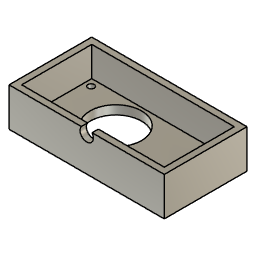
Soporte cámara individual (Parte delantera) (Autodesk Fusion 360 design; units mm, degrees)
Autodesk Fusion 360 part; units mm, degrees
sketch "Boceto1" plane through (0, 0, 0) normal (0, 0, 1) x (1, 0, 0)
  line L0 (-22.6, -11.1) -> (22.6, -11.1)
  line L1 (22.6, -11.1) -> (22.6, 11.1)
  line L2 (22.6, 11.1) -> (-22.6, 11.1)
  line L3 (-22.6, 11.1) -> (-22.6, -11.1)
  line L4 (-22.6, -11.1) -> (22.6, 11.1) construction
  line L5 (22.6, -11.1) -> (-22.6, 11.1) construction
  circle A0 centre (-5.85, 2) radius 8.15
  circle A1 centre (-20.59, 8.89) radius 1
  line L6 (0, 11.1) -> (0, -11.1) construction
  line L7 (22.6, 13.1) -> (-22.6, 13.1)
  line L8 (-22.6, 13.1) -> (-22.6, 11.1)
  line L9 (-22.6, 11.1) -> (22.6, 11.1)
  line L10 (22.6, 11.1) -> (22.6, 13.1)
  line L11 (22.6, 13.1) -> (-22.6, 11.1) construction
  line L12 (-22.6, 13.1) -> (22.6, 11.1) construction
  line L13 (22.6, -13.1) -> (-22.6, -13.1)
  line L14 (-22.6, -13.1) -> (-22.6, -11.1)
  line L15 (-22.6, -11.1) -> (22.6, -11.1)
  line L16 (22.6, -11.1) -> (22.6, -13.1)
  line L17 (22.6, -13.1) -> (-22.6, -11.1) construction
  line L18 (-22.6, -13.1) -> (22.6, -11.1) construction
  line L19 (24.6, -13.1) -> (22.6, -13.1)
  line L20 (22.6, -13.1) -> (22.6, 13.1)
  line L21 (22.6, 13.1) -> (24.6, 13.1)
  line L22 (24.6, 13.1) -> (24.6, -13.1)
  line L23 (24.6, -13.1) -> (22.6, 13.1) construction
  line L24 (22.6, -13.1) -> (24.6, 13.1) construction
  line L25 (-22.6, -13.1) -> (-24.6, -13.1)
  line L26 (-24.6, -13.1) -> (-24.6, 13.1)
  line L27 (-24.6, 13.1) -> (-22.6, 13.1)
  line L28 (-22.6, 13.1) -> (-22.6, -13.1)
  line L29 (-22.6, -13.1) -> (-24.6, 13.1) construction
  line L30 (-24.6, -13.1) -> (-22.6, 13.1) construction
  circle A2 centre (-20.59, -4.89) radius 1
  circle A3 centre (20.59, 8.89) radius 1
  circle A4 centre (20.59, -4.89) radius 1
  point P0 (0, 12.1)
  point P1 (0, -12.1)
  point P2 (23.6, 0)
  point P3 (-23.6, 0)
  dimension "d5" = 22.2
  dimension "d6" = 45.2
  dimension "d7" = 16.3
  dimension "d10" = 2
  dimension "d11" = 2.01
  dimension "d12" = 2.21
  dimension "d13" = 45.2
  dimension "d14" = 2
  dimension "d15" = 45.2
  dimension "d16" = 2
  dimension "d17" = 2
  dimension "d18" = 26.2
  dimension "d19" = 2
  dimension "d20" = 26.2
  dimension "d26" = 16.75
  dimension "d27" = 9.1
  dimension "d28" = 2
  dimension "d29" = 2.01
  dimension "d30" = 6.21
  constraint horizontal L0
  constraint perpendicular L0 L1
  constraint parallel L0 L2
  constraint parallel L1 L3
  constraint coincident L4 origin
  constraint coincident L5 origin
  constraint midpoint L2 L6.start
  constraint midpoint L0 L6.end
  constraint horizontal L7
  constraint perpendicular L7 L8
  constraint parallel L7 L9
  constraint parallel L8 L10
  constraint coincident L11 P0
  constraint coincident L12 P0
  constraint collinear L2 L9
  constraint collinear L3 L8
  constraint horizontal L13
  constraint perpendicular L13 L14
  constraint parallel L13 L15
  constraint parallel L14 L16
  constraint coincident L17 P1
  constraint coincident L18 P1
  constraint collinear L0 L15
  constraint collinear L3 L14
  constraint horizontal L19
  constraint perpendicular L19 L20
  constraint parallel L19 L21
  constraint parallel L20 L22
  constraint coincident L23 P2
  constraint coincident L24 P2
  constraint collinear L1 L20
  constraint collinear L7 L21
  constraint horizontal L25
  constraint perpendicular L25 L26
  constraint parallel L25 L27
  constraint parallel L26 L28
  constraint coincident L29 P3
  constraint coincident L30 P3
  constraint collinear L3 L28
  constraint collinear L7 L27
  constraint symmetric A1 L6 A3
  constraint symmetric L6 A2 A4
  measures "d5" distance of L0.end L1.end
  measures "d6" distance of L1.end L2.end
  measures "d7" diameter of A0
  measures "d10" diameter of A1
  measures "d11" distance of L3 A1.centre
  measures "d12" distance of L2 A1.centre
  measures "d13" distance of L2.end L1.end
  measures "d14" distance of L7.end L2.end
  measures "d15" distance of L0.start L0.end
  measures "d16" distance of L13.end L0.start
  measures "d17" distance of L7.start L21.end
  measures "d18" distance of L13.start L7.start
  measures "d19" distance of L26.end L7.end
  measures "d20" distance of L25.end L26.end
  measures "d26" distance of A0.centre L28
  measures "d27" distance of A0.centre L9
  measures "d28" diameter of A2
  measures "d29" distance of L3 A2.centre
  measures "d30" distance of L0 A2.centre
extrude "Extruir1" add sketch "Boceto1" along normal blind 2.8 contours L0 L1 L2 L3 L9 L15 L20 L28
extrude "Extruir2" add sketch "Boceto1" along normal blind 12.2 contours L3 L8 L14 L25 L26 L27 L28 | L0 L13 L14 L15 L16 L20 L28 | L1 L10 L16 L19 L20 L21 L22 | L2 L7 L8 L9 L10 L20 L28
sketch "Boceto2" plane through (0, -13.1, 0) normal (0, -1, 0) x (1, 0, 0)
  line L0 (-24.6, 0) -> (24.6, 0)
  line L1 (24.6, 0) -> (24.6, 12.2)
  line L2 (24.6, 12.2) -> (-24.6, 12.2)
  line L3 (-24.6, 12.2) -> (-24.6, 0)
  arc A0 (-1.7, 12.2) -> (1.7, 12.2) centre (0, 10.925) ccw
  line L4 (-1.7, 12.2) -> (1.7, 12.2) construction
  line L5 (0, 12.2) -> (0, 8.8) construction
  dimension "d31" = 3.4
  dimension "d32" = 3.4
  constraint coincident L2 A0.end
  constraint coincident L2 A0.start
  constraint midpoint L2 L4
  constraint midpoint L4 L5.start
  constraint midpoint A0 L5.end
  measures "d31" distance of A0.start A0.end
  measures "d32" distance of L5.start L5.end
extrude "Extruir3" cut sketch "Boceto2" against normal blind 2 contours L2 A0
equation "grosor1 = 2.8 mm"
equation "grosor2 = 2 mm"
equation "grosor3 = 7.5 mm"
equation "tolerancia = 0.1 mm"
equation "d5 = 18 mm + tolerancia * 2 + margen_cable"
equation "d6 = 45 mm + tolerancia * 2"
equation "d7 = 16.2 mm + tolerancia"
equation "d10 = 1.9 mm + tolerancia"
equation "d11 = 1.91 mm + tolerancia"
equation "d12 = 2.11 mm + tolerancia"
equation "d13 = d6"
equation "d14 = grosor2"
equation "d15 = d6"
equation "d16 = grosor2"
equation "d17 = grosor2"
equation "d18 = d5 + grosor2 * 2"
equation "d19 = grosor2"
equation "d20 = d5 + grosor2 * 2"
equation "d21 = grosor1"
equation "d23 = 10.2 mm + grosor2"
equation "margen_cable = 4 mm"
equation "d28 = d10"
equation "d29 = d11"
equation "d30 = d12 + margen_cable"
equation "d33 = -grosor2"
